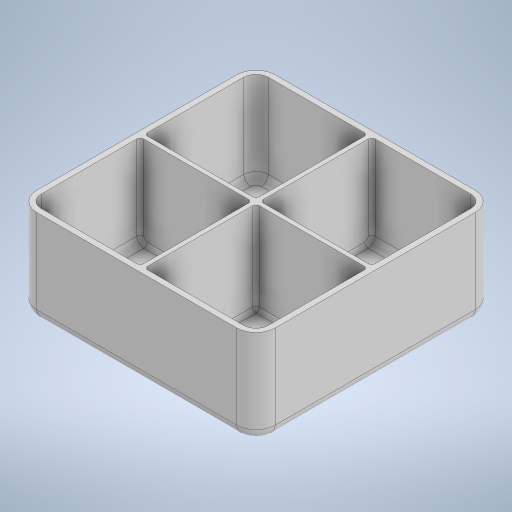
# Autodesk Inventor part: Part3
Saved by Autodesk Inventor 2023.4 (Build 274418000, 418)
## iProperties
Created: 2024-08-05
Part Number: Part3
Material: Generic
Document SubType Name: Modeling
Designer: komputer
Density: 1 g/cm^3
Appearance: Default
Author: komputer
Autodesk Inventor part; units mm, degrees
ref_plane "YZ Plane" through (0, 0, 0) normal (1, 0, 0) x (0, 1, 0)
ref_plane "XZ Plane" through (0, 0, 0) normal (0, 1, 0) x (-1, 0, 0)
ref_plane "XY Plane" through (0, 0, 0) normal (0, 0, 1) x (1, 0, 0)
sketch "Sketch1" plane through (0, 0, 0) normal (0, 1, 0) x (-1, 0, 0)
  line L0 (34, 34) -> (-34, 34)
  line L1 (-34, 34) -> (-34, -34)
  line L2 (-34, -34) -> (34, -34)
  line L3 (34, -34) -> (34, 34)
  line L4 (34, 34) -> (-34, -34) construction
  line L5 (-34, 34) -> (34, -34) construction
  point P0 (0, 0)
  dimension "d0" = 68
  dimension "d1" = 68
  constraints: 12 end point, 2 midpoint, 2 parallel, 1 horizontal, 1 perpendicular
  measures "d0" distance of L2.end L1.end
  measures "d1" distance of L1.end L0.end
extrude "Extrusion1" add sketch "Sketch1" along normal blind 1
sketch "Sketch2" plane through (0, 1, 0) normal (0, 1, 0) x (1, 0, 0)
  line L0 (34, -34) -> (34, 34) projected
  line L1 (34, 34) -> (-34, 34) projected
  line L2 (-34, 34) -> (-34, -34) projected
  line L3 (-34, -34) -> (34, -34) projected
  line L4 (-32.4, -32.4) -> (-32.4, 32.4)
  line L5 (-32.4, 32.4) -> (32.4, 32.4)
  line L6 (32.4, 32.4) -> (32.4, -32.4)
  line L7 (32.4, -32.4) -> (-32.4, -32.4)
  point P0 (0, 0)
  dimension "d4" = 1.6
  constraints: 8 end point, 3 other
  measures "d4" distance between parallel lines of L2 L4
extrude "Extrusion2" add sketch "Sketch2" along normal blind 26
fillet "Fillet1" radius 3.5 4 edges at (-32.4, 14, 32.4) (-32.4, 14, -32.4) (32.4, 14, -32.4) (32.4, 14, 32.4)
fillet "Fillet2" radius 5.5 4 edges at (34, 13.5, 34) (34, 13.5, -34) (-34, 13.5, -34) (-34, 13.5, 34)
fillet "Fillet3" radius 2 8 edges at (-31.3749, 1, 31.3749) (0, 1, 32.4) (31.3749, 1, 31.3749) (32.4, 1, 0) (31.3749, 1, -31.3749) (0, 1, -32.4) (-31.3749, 1, -31.3749) (-32.4, 1, 0)
fillet "Fillet4" radius 3 8 edges at (-32.3891, 0, 32.3891) (0, 0, 34) (32.3891, 0, 32.3891) (34, 0, 0) (32.3891, 0, -32.3891) (0, 0, -34) (-32.3891, 0, -32.3891) (-34, 0, 0)
sketch "Sketch3" plane through (0, 27, 0) normal (0, 1, 0) x (1, 0, 0)
  arc A0 (-34, -28.5) -> (-28.5, -34) centre (-28.5, -28.5) ccw projected
  line L0 (-28.5, -34) -> (28.5, -34) projected
  arc A1 (28.5, -34) -> (34, -28.5) centre (28.5, -28.5) ccw projected
  line L1 (34, -28.5) -> (34, 28.5) projected
  arc A2 (34, 28.5) -> (28.5, 34) centre (28.5, 28.5) ccw projected
  line L2 (28.5, 34) -> (-28.5, 34) projected
  arc A3 (-28.5, 34) -> (-34, 28.5) centre (-28.5, 28.5) ccw projected
  line L3 (-34, 28.5) -> (-34, -28.5) projected
  line L4 (-32.4, -28.9) -> (-32.4, 28.9) projected
  arc A4 (-28.9, 32.4) -> (-32.4, 28.9) centre (-28.9, 28.9) ccw projected
  line L5 (-28.9, 32.4) -> (28.9, 32.4) projected
  arc A5 (32.4, 28.9) -> (28.9, 32.4) centre (28.9, 28.9) ccw projected
  line L6 (32.4, 28.9) -> (32.4, -28.9) projected
  arc A6 (28.9, -32.4) -> (32.4, -28.9) centre (28.9, -28.9) ccw projected
  line L7 (28.9, -32.4) -> (-28.9, -32.4) projected
  arc A7 (-32.4, -28.9) -> (-28.9, -32.4) centre (-28.9, -28.9) ccw projected
  line L8 (-34, 28.5) -> (-34, -28.5) projected
  line L9 (-34, 0) -> (34, 0)
  line L10 (34, -28.5) -> (34, 28.5) projected
  line L11 (-28.5, -34) -> (28.5, -34) projected
  line L12 (0, -34) -> (0, 34)
  line L13 (-0.6, -34) -> (-0.6, 34)
  line L14 (0.6, -34) -> (0.6, 34)
  line L15 (-34, 0.6) -> (34, 0.6)
  line L16 (-34, -0.6) -> (34, -0.6)
  point P0 (0, 0)
  point P1 (-0.6, 0.6)
  point P2 (-32.4, 0.6)
  point P3 (-32.4, -0.6)
  point P4 (-0.6, -0.6)
  point P5 (-0.6, -32.4)
  point P6 (0.6, -32.4)
  point P7 (0.6, -0.6)
  point P8 (32.4, -0.6)
  point P9 (32.4, 0.6)
  point P10 (0.6, 0.6)
  point P11 (0.6, 32.4)
  point P12 (-0.6, 32.4)
  dimension "d11" = 0.6
  dimension "d12" = 0.6
  dimension "d13" = 0.6
  dimension "d14" = 0.6
  constraints: 12 end point, 4 midpoint, 4 parallel
  measures "d11" distance between parallel lines of L12 L13
  measures "d12" distance between parallel lines of L12 L14
  measures "d13" distance between parallel lines of L9 L15
  measures "d14" distance between parallel lines of L9 L16
extrude "Extrusion3" add sketch "Sketch3" against normal up to surface (26 mm away) contours L4 L9 L13 L16 | L13 L16 L12 L7 | L4 L15 L13 L9 | L13 L9 L12 L16 | L12 L16 L14 L7 | L13 L15 L12 L9 | L12 L9 L14 L16 | L13 L5 L12 L15 | L12 L15 L14 L9 | L14 L9 L6 L16 | L12 L5 L14 L15 | L14 L15 L6 L9
fillet "Fillet5" radius 1 4 edges at (0.6, 14, 0.6) (-0.6, 14, 0.6) (0.6, 14, -0.6) (-0.6, 14, -0.6)
fillet "Fillet6" radius 1 28 edges at (0.6, 1.5858, 31.8142) (0.6, 1, 16) (0.8929, 1, 0.8929) (16, 1, 0.6) (31.8142, 1.5858, 0.6) (32.4, 15, 0.6) (0.6, 15, 32.4) (31.8142, 1.5858, -0.6) (32.4, 15, -0.6) (0.8929, 1, -0.8929) (0.6, 1, -16) (0.6, 1.5858, -31.8142) (0.6, 15, -32.4) (16, 1, -0.6) (-0.8929, 1, -0.8929) (-0.6, 1, -16) (-0.6, 1.5858, -31.8142) (-0.6, 15, -32.4) (-31.8142, 1.5858, -0.6) (-32.4, 15, -0.6) (-16, 1, -0.6) (-31.8142, 1.5858, 0.6) (-32.4, 15, 0.6) (-0.8929, 1, 0.8929) (-0.6, 1, 16) (-0.6, 1.5858, 31.8142) (-0.6, 15, 32.4) (-16, 1, 0.6)
body "Solid1"
